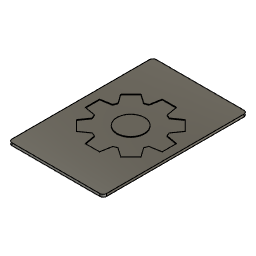
Wingspan - Automa divider (Autodesk Fusion 360 design; units mm, degrees)
Autodesk Fusion 360 part; units mm, degrees
sketch "Skizze1" plane through (0, 0, 0) normal (0, 0, 1) x (1, 0, 0)
  line L0 (0, 0) -> (57, 0)
  line L1 (57, 0) -> (57, 87)
  line L2 (57, 87) -> (0, 87)
  line L3 (0, 87) -> (0, 0)
  dimension "d1" = 57
  dimension "d2" = 87
  constraint horizontal L0
  constraint vertical L1
  constraint horizontal L2
  constraint vertical L3
  constraint coincident L0.start L3.end
  measures "d1" distance of L0.start L0.end
  measures "d2" distance of L0.start L2.end
extrude "Extrusion1" add sketch "Skizze1" along normal blind 1.75
fillet "Abrundung1" radius 2 4 edges at (0, 0, 0.875) (57, 0, 0.875) (57, 87, 0.875) (0, 87, 0.875)
sketch "Skizze2" plane through (0, 0, 1.75) normal (0, 0, 1) x (-1, 0, 0)
  arc A0 (-2, -87) -> (0, -85) centre (-2, -85) ccw
  line L0 (0, -85) -> (0, -2)
  arc A1 (0, -2) -> (-2, 0) centre (-2, -2) ccw
  line L1 (-2, 0) -> (-55, 0)
  arc A2 (-55, 0) -> (-57, -2) centre (-55, -2) ccw
  line L2 (-57, -2) -> (-57, -85)
  arc A3 (-57, -85) -> (-55, -87) centre (-55, -85) ccw
  line L3 (-55, -87) -> (-2, -87)
  line L4 (-5.5896, -49.2464) -> (-5.5896, -40.6115)
  line L5 (-5.5896, -40.6115) -> (-12.2493, -39.4747)
  spline S0 degree 3 poles (-12.2493, -39.4747) (-12.5241, -38.6458) (-12.8509, -37.8501) (-13.2393, -37.0827) knots 0 0 0 0 1 1 1 1
  line L6 (-13.2393, -37.0827) -> (-9.3316, -31.5693)
  line L7 (-9.3316, -31.5693) -> (-15.4418, -25.459)
  line L8 (-15.4418, -25.459) -> (-20.9932, -29.3904)
  spline S1 degree 3 poles (-20.9932, -29.3904) (-21.7416, -29.0162) (-22.5231, -28.7083) (-23.3331, -28.4478) knots 0 0 0 0 1 1 1 1
  line L9 (-23.3331, -28.4478) -> (-24.4794, -21.7171)
  line L10 (-24.4794, -21.7171) -> (-33.1143, -21.7171)
  line L11 (-33.1143, -21.7171) -> (-34.2747, -28.5189)
  spline S2 degree 3 poles (-34.2747, -28.5189) (-35.0515, -28.7794) (-35.7952, -29.092) (-36.5152, -29.4567) knots 0 0 0 0 1 1 1 1
  line L12 (-36.5152, -29.4567) -> (-42.1565, -25.459)
  line L13 (-42.1565, -25.459) -> (-48.2668, -31.5693)
  line L14 (-48.2668, -31.5693) -> (-44.2454, -37.2438)
  spline S3 degree 3 poles (-44.2454, -37.2438) (-44.5959, -37.9495) (-44.8801, -38.679) (-45.1359, -39.4321) knots 0 0 0 0 1 1 1 1
  line L15 (-45.1359, -39.4321) -> (-52.0087, -40.6068)
  line L16 (-52.0087, -40.6068) -> (-52.0087, -49.2464)
  line L17 (-52.0087, -49.2464) -> (-45.1311, -50.4211)
  spline S4 degree 3 poles (-45.1311, -50.4211) (-44.8801, -51.179) (-44.5911, -51.8989) (-44.2406, -52.6047) knots 0 0 0 0 1 1 1 1
  line L18 (-44.2406, -52.6047) -> (-48.262, -58.2839)
  line L19 (-48.262, -58.2839) -> (-42.1565, -64.3895)
  line L20 (-42.1565, -64.3895) -> (-36.5152, -60.3965)
  spline S5 degree 3 poles (-36.5152, -60.3965) (-35.7952, -60.7612) (-35.0515, -61.0691) (-34.2795, -61.3343) knots 0 0 0 0 1 1 1 1
  line L21 (-34.2795, -61.3343) -> (-33.1143, -68.1362)
  line L22 (-33.1143, -68.1362) -> (-24.4746, -68.1362)
  line L23 (-24.4746, -68.1362) -> (-23.3236, -61.4054)
  spline S6 degree 3 poles (-23.3236, -61.4054) (-22.5137, -61.1401) (-21.7368, -60.837) (-20.9885, -60.4628) knots 0 0 0 0 1 1 1 1
  line L24 (-20.9885, -60.4628) -> (-15.4418, -64.3942)
  line L25 (-15.4418, -64.3942) -> (-9.3316, -58.2887)
  line L26 (-9.3316, -58.2887) -> (-13.2346, -52.7752)
  spline S7 degree 3 poles (-13.2346, -52.7752) (-12.8414, -52.0079) (-12.5193, -51.2121) (-12.2446, -50.3832) knots 0 0 0 0 1 1 1 1
  line L27 (-12.2446, -50.3832) -> (-5.5896, -49.2464)
  spline S8 degree 3 poles (-28.695, -53.2157) (-33.2706, -53.2157) (-36.9841, -49.5069) (-36.9841, -44.9266) knots 0 0 0 0 1 1 1 1
  spline S9 degree 3 poles (-36.9841, -44.9266) (-36.9841, -40.351) (-33.2706, -36.6375) (-28.695, -36.6375) knots 0 0 0 0 1 1 1 1
  spline S10 degree 3 poles (-28.695, -36.6375) (-24.1146, -36.6375) (-20.4058, -40.351) (-20.4058, -44.9266) knots 0 0 0 0 1 1 1 1
  spline S11 degree 3 poles (-20.4058, -44.9266) (-20.4058, -49.5069) (-24.1194, -53.2157) (-28.695, -53.2157) knots 0 0 0 0 1 1 1 1
extrude "Extrusion2" cut sketch "Skizze2" against normal blind 0.4 contours L4 L5 S0 L6 L7 L8 S1 L9 L10 L11 S2 L12 L13 L14 S3 L15 L16 L17 S4 L18 L19 L20 S5 L21 L22 L23 S6 L24 L25 L26 S7 L27
extrude "Extrusion3" cut 1 faces at (19, 57.3333, 0) along direction (0, 0, 1) blind 0.2
extrude "Extrusion4" cut 1 faces at (19, 57.3333, 0.2) along direction (0, 0, 1) blind 0.05
